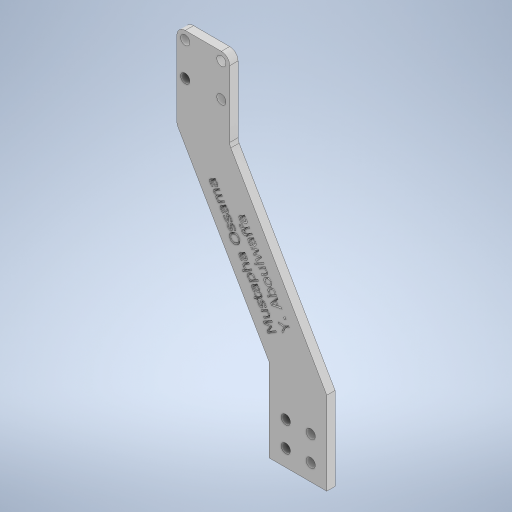
# Autodesk Inventor part: Arm
Saved by Autodesk Inventor 2023 (Build 270158000, 158)
## iProperties
Created: 2023-12-17
Part Number: Arm
Material: Generic
Document SubType Name: Modeling
Designer: Mustapha
Density: 1 g/cm^3
Appearance: Default
Author: Mustapha
Autodesk Inventor part; units mm, degrees
ref_plane "YZ Plane" through (0, 0, 0) normal (1, 0, 0) x (0, 1, 0)
ref_plane "XZ Plane" through (0, 0, 0) normal (0, 1, 0) x (-1, 0, 0)
ref_plane "XY Plane" through (0, 0, 0) normal (0, 0, 1) x (1, 0, 0)
sketch "Sketch1" plane through (0, 0, 0) normal (0, 0, 1) x (1, 0, 0)
  line L0 (0, 0) -> (-54.8483, 95)
  line L1 (-55.5181, 97.5) -> (-55.5181, 142.5)
  line L2 (-50.5181, 147.5) -> (-28.7639, 147.5)
  line L3 (-23.7639, 142.5) -> (-23.7639, 102.5)
  line L4 (-23.094, 100) -> (34.641, 0)
  line L5 (34.641, 0) -> (0, 0)
  arc A0 (-55.5181, 97.5) -> (-54.8483, 95) centre (-50.5181, 97.5) ccw
  arc A1 (-23.7639, 102.5) -> (-23.094, 100) centre (-18.7639, 102.5) ccw
  arc A2 (-23.7639, 142.5) -> (-28.7639, 147.5) centre (-28.7639, 142.5) ccw
  arc A3 (-50.5181, 147.5) -> (-55.5181, 142.5) centre (-50.5181, 142.5) ccw
  line L6 (0, 0) -> (0, -50)
  line L7 (0, -50) -> (34.641, -50)
  line L8 (34.641, -50) -> (34.641, 0)
  circle A4 centre (10, -40) radius 2.75
  circle A5 centre (25, -40) radius 2.75
  circle A6 centre (25, -25) radius 2.75
  circle A7 centre (10, -25) radius 2.75
  circle A8 centre (-50.5181, 142.5) radius 2.75
  circle A9 centre (-28.7639, 142.5) radius 2.75
  circle A10 centre (-50.5181, 122.5) radius 2.75
  circle A11 centre (-28.7639, 122.5) radius 2.75
  point P0 (-55.5181, 147.5)
  dimension "d0" = 5
  dimension "d1" = 30
  dimension "d2" = 50
  dimension "d3" = 5
  dimension "d4" = 50
  dimension "d5" = 40
  dimension "d6" = 100
  dimension "d7" = 120
  dimension "d8" = 5.5
  dimension "d11" = 15
  dimension "d18" = 15
  dimension "d23" = 10
  dimension "d24" = 10
  dimension "d25" = 5.5
  dimension "d26" = 5.5
  dimension "d29" = 20
  constraints: 18 end point, 12 centre point, 8 point on circle, 8 tangent, 5 perpendicular, 4 vertical, 2 coincident, 2 equal radius, 2 point on line, 1 horizontal, 1 parallel, 10 other
  measures "d0" radius of A0
  measures "d1" distance between parallel lines of L0 L4
  measures "d2" distance of L1.start point (-55.518, 147.5)
  measures "d3" radius of A2
  measures "d4" distance of L7.end L4.end
  measures "d5" distance of L3.start L3.end
  measures "d6" vertical distance of L4.start L4.end
  measures "d7" angle of L5 L0
  measures "d8" diameter of A4
  measures "d11" distance of A4.centre A5.centre
  measures "d18" distance of A5.centre A6.centre
  measures "d23" distance from line of L6 A7.centre
  measures "d24" distance from line of L7 A4.centre
  measures "d25" diameter of A8
  measures "d26" diameter of A9
  measures "d29" distance of A8.centre A10.centre
extrude "Extrusion1" add sketch "Sketch1" along normal blind 5
sketch "Sketch2" plane through (0, 0, 5) normal (0, 0, 1) x (1, 0, 0)
  line L0 (-0.614, 13.88) -> (-77.0258, 141.9094) construction
  line L1 (-77.0258, 141.9094) -> (-33.2435, 168.0399) construction
  line L2 (-33.2435, 168.0399) -> (43.1682, 40.0105) construction
  line L3 (43.1682, 40.0105) -> (-0.614, 13.88) construction
  line L4 (1.5283, 22.5197) -> (1.9769, 21.7682)
  line L5 (1.9769, 21.7682) -> (-2.4613, 19.1193)
  line L6 (-2.4613, 19.1193) -> (1.4369, 19.4471)
  line L7 (1.4369, 19.4471) -> (1.7085, 18.992)
  line L8 (1.7085, 18.992) -> (-0.4355, 15.7249)
  line L9 (-0.4355, 15.7249) -> (4.0027, 18.3738)
  line L10 (4.0027, 18.3738) -> (4.4239, 17.6681)
  line L11 (4.4239, 17.6681) -> (-0.7283, 14.5932)
  line L12 (-0.7283, 14.5932) -> (-1.3413, 15.6203)
  line L13 (-1.3413, 15.6203) -> (0.6823, 18.7476)
  line L14 (0.6823, 18.7476) -> (-3.0009, 18.4009)
  line L15 (-3.0009, 18.4009) -> (-3.6238, 19.4447)
  line L16 (-3.6238, 19.4447) -> (1.5283, 22.5197)
  line L17 (-1.1006, 26.9245) -> (-0.6745, 26.2105)
  line L18 (-0.6745, 26.2105) -> (-1.1004, 25.9564)
  spline S0 degree 2 poles (-1.1004, 25.9564) (-0.6405, 25.7835) (-0.0127, 25.3484) (0.2041, 24.9852) knots 0 0 0 1 2 2 2
  spline S1 degree 2 poles (0.2041, 24.9852) (0.371, 24.7055) (0.4956, 24.1173) (0.4257, 23.8264) knots 0 0 0 1 2 2 2
  spline S2 degree 2 poles (0.4257, 23.8264) (0.3558, 23.5356) (-0.0716, 23.0087) (-0.464, 22.7745) knots 0 0 0 1 2 2 2
  line L19 (-0.464, 22.7745) -> (-2.9733, 21.2769)
  line L20 (-2.9733, 21.2769) -> (-3.3994, 21.9908)
  line L21 (-3.3994, 21.9908) -> (-1.1949, 23.3065)
  spline S3 degree 2 poles (-1.1949, 23.3065) (-0.886, 23.4909) (-0.5109, 23.7828) (-0.4129, 23.9601) knots 0 0 0 1 2 2 2
  spline S4 degree 2 poles (-0.4129, 23.9601) (-0.3149, 24.1375) (-0.3566, 24.5204) (-0.5235, 24.8001) knots 0 0 0 1 2 2 2
  spline S5 degree 2 poles (-0.5235, 24.8001) (-0.6805, 25.0631) (-1.3082, 25.4982) (-1.6515, 25.6274) knots 0 0 0 1 2 2 2
  line L22 (-1.6515, 25.6274) -> (-4.5407, 23.9031)
  line L23 (-4.5407, 23.9031) -> (-4.9668, 24.617)
  line L24 (-4.9668, 24.617) -> (-1.1006, 26.9245)
  spline S6 degree 2 poles (-2.312, 29.1629) (-2.0578, 28.737) (-1.823, 27.8693) (-1.7954, 27.5573) knots 0 0 0 1 2 2 2
  line L25 (-1.7954, 27.5573) -> (-2.526, 27.1213)
  line L26 (-2.526, 27.1213) -> (-2.5485, 27.1588)
  spline S7 degree 2 poles (-2.5485, 27.1588) (-2.5365, 27.2906) (-2.5249, 27.6316) (-2.5593, 27.8885) knots 0 0 0 1 2 2 2
  spline S8 degree 2 poles (-2.5593, 27.8885) (-2.5896, 28.1196) (-2.7343, 28.6277) (-2.8739, 28.8615) knots 0 0 0 1 2 2 2
  spline S9 degree 2 poles (-2.8739, 28.8615) (-2.976, 29.0327) (-3.2829, 29.3762) (-3.3945, 29.4398) knots 0 0 0 1 2 2 2
  spline S10 degree 2 poles (-3.3945, 29.4398) (-3.5536, 29.526) (-3.8029, 29.5358) (-3.9866, 29.4262) knots 0 0 0 1 2 2 2
  spline S11 degree 2 poles (-3.9866, 29.4262) (-4.2204, 29.2866) (-4.2898, 28.8715) (-4.1573, 28.4693) knots 0 0 0 1 2 2 2
  spline S12 degree 2 poles (-4.1573, 28.4693) (-4.1085, 28.3116) (-3.9261, 27.8258) (-3.8599, 27.6105) knots 0 0 0 1 2 2 2
  spline S13 degree 2 poles (-3.8599, 27.6105) (-3.7003, 27.049) (-3.9706, 26.2874) (-4.3547, 26.0582) knots 0 0 0 1 2 2 2
  spline S14 degree 2 poles (-4.3547, 26.0582) (-4.8766, 25.7467) (-6.0504, 26.2239) (-6.479, 26.942) knots 0 0 0 1 2 2 2
  spline S15 degree 2 poles (-6.479, 26.942) (-6.6883, 27.2928) (-6.9583, 28.1056) (-6.9817, 28.42) knots 0 0 0 1 2 2 2
  line L27 (-6.9817, 28.42) -> (-6.2845, 28.8361)
  line L28 (-6.2845, 28.8361) -> (-6.262, 28.7986)
  spline S16 degree 2 poles (-6.262, 28.7986) (-6.298, 28.4034) (-6.1264, 27.5941) (-5.9221, 27.2518) knots 0 0 0 1 2 2 2
  spline S17 degree 2 poles (-5.9221, 27.2518) (-5.7128, 26.9011) (-5.1498, 26.5745) (-4.8785, 26.7365) knots 0 0 0 1 2 2 2
  spline S18 degree 2 poles (-4.8785, 26.7365) (-4.6321, 26.8835) (-4.5661, 27.3137) (-4.6803, 27.6758) knots 0 0 0 1 2 2 2
  spline S19 degree 2 poles (-4.6803, 27.6758) (-4.7399, 27.8611) (-4.8965, 28.2942) (-4.9802, 28.5387) knots 0 0 0 1 2 2 2
  spline S20 degree 2 poles (-4.9802, 28.5387) (-5.1532, 29.0753) (-4.9404, 29.8478) (-4.5104, 30.1045) knots 0 0 0 1 2 2 2
  spline S21 degree 2 poles (-4.5104, 30.1045) (-4.2599, 30.254) (-3.6877, 30.301) (-3.4003, 30.1894) knots 0 0 0 1 2 2 2
  spline S22 degree 2 poles (-3.4003, 30.1894) (-3.0921, 30.062) (-2.5711, 29.5971) (-2.312, 29.1629) knots 0 0 0 1 2 2 2
  spline S23 degree 2 poles (-4.4866, 32.7686) (-4.1378, 32.1841) (-4.3519, 31.1673) (-5.0075, 30.7761) knots 0 0 0 1 2 2 2
  line L29 (-5.0075, 30.7761) -> (-7.1493, 29.4977)
  line L30 (-7.1493, 29.4977) -> (-6.8603, 29.0134)
  line L31 (-6.8603, 29.0134) -> (-7.3988, 28.692)
  line L32 (-7.3988, 28.692) -> (-7.6879, 29.1763)
  line L33 (-7.6879, 29.1763) -> (-8.7985, 28.5135)
  line L34 (-8.7985, 28.5135) -> (-9.2246, 29.2274)
  line L35 (-9.2246, 29.2274) -> (-8.114, 29.8903)
  line L36 (-8.114, 29.8903) -> (-8.8989, 31.2054)
  line L37 (-8.8989, 31.2054) -> (-8.3604, 31.5269)
  line L38 (-8.3604, 31.5269) -> (-7.5754, 30.2117)
  line L39 (-7.5754, 30.2117) -> (-5.7342, 31.3106)
  spline S24 degree 2 poles (-5.7342, 31.3106) (-5.4419, 31.485) (-5.1329, 31.6978) (-5.0424, 31.8594) knots 0 0 0 1 2 2 2
  spline S25 degree 2 poles (-5.0424, 31.8594) (-4.9587, 31.9942) (-5.0096, 32.3546) (-5.1591, 32.6051) knots 0 0 0 1 2 2 2
  spline S26 degree 2 poles (-5.1591, 32.6051) (-5.2613, 32.7763) (-5.5542, 33.0488) (-5.6258, 33.1023) knots 0 0 0 1 2 2 2
  line L40 (-5.6258, 33.1023) -> (-5.6507, 33.1441)
  line L41 (-5.6507, 33.1441) -> (-5.0661, 33.493)
  spline S27 degree 2 poles (-5.0661, 33.493) (-4.8964, 33.3225) (-4.5913, 32.944) (-4.4866, 32.7686) knots 0 0 0 1 2 2 2
  spline S28 degree 2 poles (-7.1713, 36.1663) (-7.0605, 36.1135) (-6.6773, 35.9458) (-6.5324, 35.8454) knots 0 0 0 1 2 2 2
  spline S29 degree 2 poles (-6.5324, 35.8454) (-6.3284, 35.7123) (-6.0206, 35.4148) (-5.8312, 35.0974) knots 0 0 0 1 2 2 2
  spline S30 degree 2 poles (-5.8312, 35.0974) (-5.6742, 34.8344) (-5.5722, 34.2555) (-5.6279, 33.9787) knots 0 0 0 1 2 2 2
  spline S31 degree 2 poles (-5.6279, 33.9787) (-5.6844, 33.7129) (-6.0299, 33.2292) (-6.2887, 33.0747) knots 0 0 0 1 2 2 2
  spline S32 degree 2 poles (-6.2887, 33.0747) (-6.6896, 32.8355) (-7.4792, 32.8682) (-7.8837, 33.176) knots 0 0 0 1 2 2 2
  spline S33 degree 2 poles (-7.8837, 33.176) (-8.2458, 33.4412) (-8.9391, 34.3467) (-9.3048, 34.8929) knots 0 0 0 1 2 2 2
  line L42 (-9.3048, 34.8929) -> (-9.43, 34.8182)
  spline S34 degree 2 poles (-9.43, 34.8182) (-9.6555, 34.6836) (-9.8455, 34.3663) (-9.8426, 34.1812) knots 0 0 0 1 2 2 2
  spline S35 degree 2 poles (-9.8426, 34.1812) (-9.8397, 33.9961) (-9.6531, 33.5695) (-9.5285, 33.3608) knots 0 0 0 1 2 2 2
  spline S36 degree 2 poles (-9.5285, 33.3608) (-9.3815, 33.1144) (-8.8492, 32.5262) (-8.5204, 32.2694) knots 0 0 0 1 2 2 2
  line L43 (-8.5204, 32.2694) -> (-8.4955, 32.2276)
  line L44 (-8.4955, 32.2276) -> (-9.1593, 31.8314)
  spline S37 degree 2 poles (-9.1593, 31.8314) (-9.3265, 31.9978) (-9.8929, 32.662) (-10.1096, 33.0253) knots 0 0 0 1 2 2 2
  spline S38 degree 2 poles (-10.1096, 33.0253) (-10.3688, 33.4595) (-10.6024, 34.1355) (-10.5841, 34.4748) knots 0 0 0 1 2 2 2
  spline S39 degree 2 poles (-10.5841, 34.4748) (-10.5625, 34.7991) (-10.1943, 35.3303) (-9.8311, 35.5471) knots 0 0 0 1 2 2 2
  line L45 (-9.8311, 35.5471) -> (-7.1882, 37.1244)
  line L46 (-7.1882, 37.1244) -> (-6.7621, 36.4105)
  line L47 (-6.7621, 36.4105) -> (-7.1713, 36.1663)
  line L48 (-7.714, 35.8423) -> (-8.7871, 35.2019)
  spline S40 degree 2 poles (-8.7871, 35.2019) (-8.6142, 34.9597) (-8.0797, 34.2255) (-7.8684, 34.0232) knots 0 0 0 1 2 2 2
  spline S41 degree 2 poles (-7.8684, 34.0232) (-7.6196, 33.7866) (-7.068, 33.6119) (-6.7757, 33.7863) knots 0 0 0 1 2 2 2
  spline S42 degree 2 poles (-6.7757, 33.7863) (-6.4417, 33.9856) (-6.3477, 34.5967) (-6.5845, 34.9933) knots 0 0 0 1 2 2 2
  spline S43 degree 2 poles (-6.5845, 34.9933) (-6.7863, 35.3315) (-7.3758, 35.7214) (-7.714, 35.8423) knots 0 0 0 1 2 2 2
  spline S44 degree 2 poles (-11.9518, 40.476) (-10.9831, 41.0541) (-9.2336, 40.7223) (-8.7701, 39.9457) knots 0 0 0 1 2 2 2
  spline S45 degree 2 poles (-8.7701, 39.9457) (-8.5833, 39.6326) (-8.4253, 39.0644) (-8.4111, 38.7275) knots 0 0 0 1 2 2 2
  line L49 (-8.4111, 38.7275) -> (-6.7911, 39.6943)
  line L50 (-6.7911, 39.6943) -> (-6.365, 38.9803)
  line L51 (-6.365, 38.9803) -> (-11.6549, 35.8232)
  line L52 (-11.6549, 35.8232) -> (-12.0811, 36.5371)
  line L53 (-12.0811, 36.5371) -> (-11.6761, 36.7788)
  spline S46 degree 2 poles (-11.6761, 36.7788) (-12.0568, 36.914) (-12.7353, 37.3867) (-12.9646, 37.7708) knots 0 0 0 1 2 2 2
  spline S47 degree 2 poles (-12.9646, 37.7708) (-13.4007, 38.5015) (-12.8369, 39.9477) (-11.9518, 40.476) knots 0 0 0 1 2 2 2
  spline S48 degree 2 poles (-11.4356, 39.7819) (-12.0994, 39.3856) (-12.5535, 38.4861) (-12.242, 37.9642) knots 0 0 0 1 2 2 2
  spline S49 degree 2 poles (-12.242, 37.9642) (-12.0626, 37.6636) (-11.4774, 37.2428) (-11.1333, 37.1028) knots 0 0 0 1 2 2 2
  line L54 (-11.1333, 37.1028) -> (-8.9372, 38.4135)
  spline S50 degree 2 poles (-8.9372, 38.4135) (-8.983, 38.7655) (-9.1304, 39.2211) (-9.2849, 39.48) knots 0 0 0 1 2 2 2
  spline S51 degree 2 poles (-9.2849, 39.48) (-9.6163, 40.0353) (-10.7258, 40.2055) (-11.4356, 39.7819) knots 0 0 0 1 2 2 2
  line L55 (-12.3513, 45.7753) -> (-11.9252, 45.0614)
  line L56 (-11.9252, 45.0614) -> (-14.1297, 43.7457)
  spline S52 degree 2 poles (-14.1297, 43.7457) (-14.3969, 43.5862) (-14.8213, 43.2537) (-14.9117, 43.0921) knots 0 0 0 1 2 2 2
  spline S53 degree 2 poles (-14.9117, 43.0921) (-15.0055, 42.9172) (-14.9606, 42.5193) (-14.8011, 42.2521) knots 0 0 0 1 2 2 2
  spline S54 degree 2 poles (-14.8011, 42.2521) (-14.6417, 41.9849) (-14.0439, 41.5716) (-13.6732, 41.4248) knots 0 0 0 1 2 2 2
  line L57 (-13.6732, 41.4248) -> (-10.784, 43.1492)
  line L58 (-10.784, 43.1492) -> (-10.3579, 42.4352)
  line L59 (-10.3579, 42.4352) -> (-15.7396, 39.2232)
  line L60 (-15.7396, 39.2232) -> (-16.1657, 39.9372)
  line L61 (-16.1657, 39.9372) -> (-14.2201, 41.0984)
  spline S55 degree 2 poles (-14.2201, 41.0984) (-14.675, 41.2629) (-15.3219, 41.7205) (-15.5287, 42.067) knots 0 0 0 1 2 2 2
  spline S56 degree 2 poles (-15.5287, 42.067) (-15.9025, 42.6933) (-15.5746, 43.8516) (-14.8606, 44.2777) knots 0 0 0 1 2 2 2
  line L62 (-14.8606, 44.2777) -> (-12.3513, 45.7753)
  spline S57 degree 2 poles (-14.7739, 48.9047) (-14.6631, 48.8519) (-14.28, 48.6842) (-14.1351, 48.5838) knots 0 0 0 1 2 2 2
  spline S58 degree 2 poles (-14.1351, 48.5838) (-13.9311, 48.4507) (-13.6233, 48.1532) (-13.4339, 47.8359) knots 0 0 0 1 2 2 2
  spline S59 degree 2 poles (-13.4339, 47.8359) (-13.2769, 47.5728) (-13.1749, 46.9939) (-13.2305, 46.7172) knots 0 0 0 1 2 2 2
  spline S60 degree 2 poles (-13.2305, 46.7172) (-13.287, 46.4513) (-13.6325, 45.9676) (-13.8914, 45.8131) knots 0 0 0 1 2 2 2
  spline S61 degree 2 poles (-13.8914, 45.8131) (-14.2922, 45.5739) (-15.0818, 45.6066) (-15.4864, 45.9144) knots 0 0 0 1 2 2 2
  spline S62 degree 2 poles (-15.4864, 45.9144) (-15.8485, 46.1796) (-16.5418, 47.0851) (-16.9074, 47.6313) knots 0 0 0 1 2 2 2
  line L63 (-16.9074, 47.6313) -> (-17.0327, 47.5566)
  spline S63 degree 2 poles (-17.0327, 47.5566) (-17.2582, 47.422) (-17.4482, 47.1048) (-17.4453, 46.9196) knots 0 0 0 1 2 2 2
  spline S64 degree 2 poles (-17.4453, 46.9196) (-17.4424, 46.7345) (-17.2557, 46.308) (-17.1312, 46.0992) knots 0 0 0 1 2 2 2
  spline S65 degree 2 poles (-17.1312, 46.0992) (-16.9841, 45.8529) (-16.4518, 45.2646) (-16.1231, 45.0078) knots 0 0 0 1 2 2 2
  line L64 (-16.1231, 45.0078) -> (-16.0981, 44.9661)
  line L65 (-16.0981, 44.9661) -> (-16.762, 44.5699)
  spline S66 degree 2 poles (-16.762, 44.5699) (-16.9292, 44.7362) (-17.4955, 45.4004) (-17.7123, 45.7637) knots 0 0 0 1 2 2 2
  spline S67 degree 2 poles (-17.7123, 45.7637) (-17.9715, 46.1979) (-18.205, 46.8739) (-18.1867, 47.2132) knots 0 0 0 1 2 2 2
  spline S68 degree 2 poles (-18.1867, 47.2132) (-18.1651, 47.5375) (-17.797, 48.0687) (-17.4338, 48.2855) knots 0 0 0 1 2 2 2
  line L66 (-17.4338, 48.2855) -> (-14.7909, 49.8628)
  line L67 (-14.7909, 49.8628) -> (-14.3648, 49.1489)
  line L68 (-14.3648, 49.1489) -> (-14.7739, 48.9047)
  line L69 (-15.3167, 48.5807) -> (-16.3897, 47.9403)
  spline S69 degree 2 poles (-16.3897, 47.9403) (-16.2168, 47.6981) (-15.6824, 46.9639) (-15.471, 46.7616) knots 0 0 0 1 2 2 2
  spline S70 degree 2 poles (-15.471, 46.7616) (-15.2223, 46.525) (-14.6707, 46.3503) (-14.3784, 46.5247) knots 0 0 0 1 2 2 2
  spline S71 degree 2 poles (-14.3784, 46.5247) (-14.0444, 46.7241) (-13.9504, 47.3351) (-14.1871, 47.7317) knots 0 0 0 1 2 2 2
  spline S72 degree 2 poles (-14.1871, 47.7317) (-14.389, 48.0699) (-14.9784, 48.4599) (-15.3167, 48.5807) knots 0 0 0 1 2 2 2
  spline S73 degree 2 poles (-23.8322, 54.642) (-23.6817, 55.1678) (-22.894, 56.1249) (-22.251, 56.5087) knots 0 0 0 1 2 2 2
  spline S74 degree 2 poles (-22.251, 56.5087) (-21.6247, 56.8824) (-20.4008, 57.1373) (-19.8616, 57.0117) knots 0 0 0 1 2 2 2
  spline S75 degree 2 poles (-19.8616, 57.0117) (-19.2957, 56.8795) (-18.4027, 56.1611) (-18.0712, 55.6058) knots 0 0 0 1 2 2 2
  spline S76 degree 2 poles (-18.0712, 55.6058) (-17.7274, 55.0297) (-17.5316, 53.8951) (-17.6812, 53.3585) knots 0 0 0 1 2 2 2
  spline S77 degree 2 poles (-17.6812, 53.3585) (-17.8292, 52.8285) (-18.6261, 51.8772) (-19.2608, 51.4985) knots 0 0 0 1 2 2 2
  spline S78 degree 2 poles (-19.2608, 51.4985) (-19.9079, 51.1122) (-21.1051, 50.879) (-21.6543, 50.9929) knots 0 0 0 1 2 2 2
  spline S79 degree 2 poles (-21.6543, 50.9929) (-22.191, 51.1142) (-23.0991, 51.8293) (-23.4405, 52.4013) knots 0 0 0 1 2 2 2
  spline S80 degree 2 poles (-23.4405, 52.4013) (-23.7844, 52.9775) (-23.9702, 54.1236) (-23.8322, 54.642) knots 0 0 0 1 2 2 2
  spline S81 degree 2 poles (-21.7825, 55.7237) (-22.2919, 55.4197) (-22.9365, 54.7066) (-23.0633, 54.3308) knots 0 0 0 1 2 2 2
  spline S82 degree 2 poles (-23.0633, 54.3308) (-23.1959, 53.9459) (-23.0844, 53.1518) (-22.8476, 52.7551) knots 0 0 0 1 2 2 2
  spline S83 degree 2 poles (-22.8476, 52.7551) (-22.6034, 52.346) (-21.9808, 51.8909) (-21.5632, 51.8174) knots 0 0 0 1 2 2 2
  spline S84 degree 2 poles (-21.5632, 51.8174) (-21.1656, 51.7489) (-20.2303, 51.9844) (-19.7292, 52.2834) knots 0 0 0 1 2 2 2
  spline S85 degree 2 poles (-19.7292, 52.2834) (-18.7147, 52.8889) (-18.1957, 54.4671) (-18.6641, 55.252) knots 0 0 0 1 2 2 2
  spline S86 degree 2 poles (-18.6641, 55.252) (-19.1351, 56.0411) (-20.768, 56.3293) (-21.7825, 55.7237) knots 0 0 0 1 2 2 2
  spline S87 degree 2 poles (-20.7268, 60.0174) (-20.4727, 59.5915) (-20.2379, 58.7237) (-20.2102, 58.4118) knots 0 0 0 1 2 2 2
  line L70 (-20.2102, 58.4118) -> (-20.9409, 57.9757)
  line L71 (-20.9409, 57.9757) -> (-20.9633, 58.0133)
  spline S88 degree 2 poles (-20.9633, 58.0133) (-20.9513, 58.145) (-20.9397, 58.486) (-20.9741, 58.743) knots 0 0 0 1 2 2 2
  spline S89 degree 2 poles (-20.9741, 58.743) (-21.0044, 58.974) (-21.1492, 59.4822) (-21.2887, 59.716) knots 0 0 0 1 2 2 2
  spline S90 degree 2 poles (-21.2887, 59.716) (-21.3909, 59.8872) (-21.6978, 60.2306) (-21.8094, 60.2942) knots 0 0 0 1 2 2 2
  spline S91 degree 2 poles (-21.8094, 60.2942) (-21.9684, 60.3805) (-22.2177, 60.3902) (-22.4015, 60.2806) knots 0 0 0 1 2 2 2
  spline S92 degree 2 poles (-22.4015, 60.2806) (-22.6353, 60.1411) (-22.7046, 59.726) (-22.5721, 59.3237) knots 0 0 0 1 2 2 2
  spline S93 degree 2 poles (-22.5721, 59.3237) (-22.5233, 59.166) (-22.341, 58.6803) (-22.2748, 58.465) knots 0 0 0 1 2 2 2
  spline S94 degree 2 poles (-22.2748, 58.465) (-22.1152, 57.9034) (-22.3854, 57.1419) (-22.7696, 56.9126) knots 0 0 0 1 2 2 2
  spline S95 degree 2 poles (-22.7696, 56.9126) (-23.2914, 56.6012) (-24.4653, 57.0784) (-24.8939, 57.7965) knots 0 0 0 1 2 2 2
  spline S96 degree 2 poles (-24.8939, 57.7965) (-25.1032, 58.1472) (-25.3731, 58.96) (-25.3966, 59.2744) knots 0 0 0 1 2 2 2
  line L72 (-25.3966, 59.2744) -> (-24.6993, 59.6906)
  line L73 (-24.6993, 59.6906) -> (-24.6769, 59.653)
  spline S97 degree 2 poles (-24.6769, 59.653) (-24.7128, 59.2578) (-24.5413, 58.4486) (-24.3369, 58.1062) knots 0 0 0 1 2 2 2
  spline S98 degree 2 poles (-24.3369, 58.1062) (-24.1276, 57.7555) (-23.5647, 57.429) (-23.2933, 57.591) knots 0 0 0 1 2 2 2
  spline S99 degree 2 poles (-23.2933, 57.591) (-23.047, 57.738) (-22.9809, 58.1681) (-23.0952, 58.5303) knots 0 0 0 1 2 2 2
  spline S100 degree 2 poles (-23.0952, 58.5303) (-23.1548, 58.7155) (-23.3113, 59.1487) (-23.395, 59.3932) knots 0 0 0 1 2 2 2
  spline S101 degree 2 poles (-23.395, 59.3932) (-23.568, 59.9298) (-23.3553, 60.7023) (-22.9252, 60.9589) knots 0 0 0 1 2 2 2
  spline S102 degree 2 poles (-22.9252, 60.9589) (-22.6747, 61.1084) (-22.1026, 61.1555) (-21.8151, 61.0439) knots 0 0 0 1 2 2 2
  spline S103 degree 2 poles (-21.8151, 61.0439) (-21.5069, 60.9164) (-20.986, 60.4516) (-20.7268, 60.0174) knots 0 0 0 1 2 2 2
  spline S104 degree 2 poles (-22.8025, 63.4953) (-22.5484, 63.0694) (-22.3136, 62.2016) (-22.286, 61.8897) knots 0 0 0 1 2 2 2
  line L74 (-22.286, 61.8897) -> (-23.0166, 61.4536)
  line L75 (-23.0166, 61.4536) -> (-23.039, 61.4912)
  spline S105 degree 2 poles (-23.039, 61.4912) (-23.0271, 61.6229) (-23.0154, 61.964) (-23.0498, 62.2209) knots 0 0 0 1 2 2 2
  spline S106 degree 2 poles (-23.0498, 62.2209) (-23.0802, 62.4519) (-23.2249, 62.9601) (-23.3644, 63.1939) knots 0 0 0 1 2 2 2
  spline S107 degree 2 poles (-23.3644, 63.1939) (-23.4666, 63.3651) (-23.7735, 63.7085) (-23.8851, 63.7721) knots 0 0 0 1 2 2 2
  spline S108 degree 2 poles (-23.8851, 63.7721) (-24.0442, 63.8584) (-24.2935, 63.8682) (-24.4772, 63.7585) knots 0 0 0 1 2 2 2
  spline S109 degree 2 poles (-24.4772, 63.7585) (-24.711, 63.619) (-24.7803, 63.2039) (-24.6479, 62.8016) knots 0 0 0 1 2 2 2
  spline S110 degree 2 poles (-24.6479, 62.8016) (-24.599, 62.6439) (-24.4167, 62.1582) (-24.3505, 61.9429) knots 0 0 0 1 2 2 2
  spline S111 degree 2 poles (-24.3505, 61.9429) (-24.1909, 61.3813) (-24.4612, 60.6198) (-24.8453, 60.3905) knots 0 0 0 1 2 2 2
  spline S112 degree 2 poles (-24.8453, 60.3905) (-25.3672, 60.0791) (-26.541, 60.5563) (-26.9696, 61.2744) knots 0 0 0 1 2 2 2
  spline S113 degree 2 poles (-26.9696, 61.2744) (-27.1789, 61.6251) (-27.4488, 62.4379) (-27.4723, 62.7524) knots 0 0 0 1 2 2 2
  line L76 (-27.4723, 62.7524) -> (-26.775, 63.1685)
  line L77 (-26.775, 63.1685) -> (-26.7526, 63.1309)
  spline S114 degree 2 poles (-26.7526, 63.1309) (-26.7885, 62.7358) (-26.617, 61.9265) (-26.4127, 61.5841) knots 0 0 0 1 2 2 2
  spline S115 degree 2 poles (-26.4127, 61.5841) (-26.2033, 61.2334) (-25.6404, 60.9069) (-25.369, 61.0689) knots 0 0 0 1 2 2 2
  spline S116 degree 2 poles (-25.369, 61.0689) (-25.1227, 61.2159) (-25.0566, 61.646) (-25.1709, 62.0082) knots 0 0 0 1 2 2 2
  spline S117 degree 2 poles (-25.1709, 62.0082) (-25.2305, 62.1934) (-25.3871, 62.6266) (-25.4707, 62.8711) knots 0 0 0 1 2 2 2
  spline S118 degree 2 poles (-25.4707, 62.8711) (-25.6437, 63.4077) (-25.431, 64.1802) (-25.0009, 64.4368) knots 0 0 0 1 2 2 2
  spline S119 degree 2 poles (-25.0009, 64.4368) (-24.7504, 64.5864) (-24.1783, 64.6334) (-23.8909, 64.5218) knots 0 0 0 1 2 2 2
  spline S120 degree 2 poles (-23.8909, 64.5218) (-23.5826, 64.3943) (-23.0617, 63.9295) (-22.8025, 63.4953) knots 0 0 0 1 2 2 2
  spline S121 degree 2 poles (-26.1069, 67.8933) (-25.9961, 67.8405) (-25.6129, 67.6728) (-25.4681, 67.5724) knots 0 0 0 1 2 2 2
  spline S122 degree 2 poles (-25.4681, 67.5724) (-25.2641, 67.4394) (-24.9563, 67.1418) (-24.7669, 66.8245) knots 0 0 0 1 2 2 2
  spline S123 degree 2 poles (-24.7669, 66.8245) (-24.6099, 66.5615) (-24.5078, 65.9825) (-24.5635, 65.7058) knots 0 0 0 1 2 2 2
  spline S124 degree 2 poles (-24.5635, 65.7058) (-24.62, 65.4399) (-24.9655, 64.9563) (-25.2244, 64.8018) knots 0 0 0 1 2 2 2
  spline S125 degree 2 poles (-25.2244, 64.8018) (-25.6252, 64.5625) (-26.4148, 64.5952) (-26.8193, 64.9031) knots 0 0 0 1 2 2 2
  spline S126 degree 2 poles (-26.8193, 64.9031) (-27.1815, 65.1682) (-27.8748, 66.0738) (-28.2404, 66.62) knots 0 0 0 1 2 2 2
  line L78 (-28.2404, 66.62) -> (-28.3657, 66.5452)
  spline S127 degree 2 poles (-28.3657, 66.5452) (-28.5911, 66.4107) (-28.7812, 66.0934) (-28.7783, 65.9083) knots 0 0 0 1 2 2 2
  spline S128 degree 2 poles (-28.7783, 65.9083) (-28.7754, 65.7231) (-28.5887, 65.2966) (-28.4641, 65.0878) knots 0 0 0 1 2 2 2
  spline S129 degree 2 poles (-28.4641, 65.0878) (-28.3171, 64.8415) (-27.7848, 64.2532) (-27.456, 63.9965) knots 0 0 0 1 2 2 2
  line L79 (-27.456, 63.9965) -> (-27.4311, 63.9547)
  line L80 (-27.4311, 63.9547) -> (-28.095, 63.5585)
  spline S130 degree 2 poles (-28.095, 63.5585) (-28.2622, 63.7248) (-28.8285, 64.3891) (-29.0453, 64.7523) knots 0 0 0 1 2 2 2
  spline S131 degree 2 poles (-29.0453, 64.7523) (-29.3044, 65.1865) (-29.538, 65.8625) (-29.5197, 66.2019) knots 0 0 0 1 2 2 2
  spline S132 degree 2 poles (-29.5197, 66.2019) (-29.4981, 66.5262) (-29.13, 67.0573) (-28.7667, 67.2741) knots 0 0 0 1 2 2 2
  line L81 (-28.7667, 67.2741) -> (-26.1239, 68.8515)
  line L82 (-26.1239, 68.8515) -> (-25.6977, 68.1375)
  line L83 (-25.6977, 68.1375) -> (-26.1069, 67.8933)
  line L84 (-26.6497, 67.5694) -> (-27.7227, 66.929)
  spline S133 degree 2 poles (-27.7227, 66.929) (-27.5498, 66.6867) (-27.0154, 65.9525) (-26.804, 65.7502) knots 0 0 0 1 2 2 2
  spline S134 degree 2 poles (-26.804, 65.7502) (-26.5552, 65.5137) (-26.0036, 65.3389) (-25.7114, 65.5134) knots 0 0 0 1 2 2 2
  spline S135 degree 2 poles (-25.7114, 65.5134) (-25.3774, 65.7127) (-25.2834, 66.3237) (-25.5201, 66.7204) knots 0 0 0 1 2 2 2
  spline S136 degree 2 poles (-25.5201, 66.7204) (-25.7219, 67.0585) (-26.3114, 67.4485) (-26.6497, 67.5694) knots 0 0 0 1 2 2 2
  line L85 (-29.605, 74.6842) -> (-31.8429, 73.3485)
  spline S137 degree 2 poles (-31.8429, 73.3485) (-32.1101, 73.189) (-32.5378, 72.8715) (-32.6207, 72.7258) knots 0 0 0 1 2 2 2
  spline S138 degree 2 poles (-32.6207, 72.7258) (-32.7111, 72.5642) (-32.6777, 72.2047) (-32.5332, 71.9626) knots 0 0 0 1 2 2 2
  spline S139 degree 2 poles (-32.5332, 71.9626) (-32.4036, 71.7455) (-31.8533, 71.3831) (-31.4575, 71.2513) knots 0 0 0 1 2 2 2
  spline S140 degree 2 poles (-31.4575, 71.2513) (-31.4016, 71.2903) (-31.2462, 71.4001) (-31.1376, 71.4648) knots 0 0 0 1 2 2 2
  line L86 (-31.1376, 71.4648) -> (-28.5908, 72.9849)
  line L87 (-28.5908, 72.9849) -> (-28.1647, 72.2709)
  line L88 (-28.1647, 72.2709) -> (-30.4026, 70.9353)
  spline S141 degree 2 poles (-30.4026, 70.9353) (-30.6698, 70.7758) (-31.0975, 70.4583) (-31.1804, 70.3125) knots 0 0 0 1 2 2 2
  spline S142 degree 2 poles (-31.1804, 70.3125) (-31.2708, 70.151) (-31.2374, 69.7915) (-31.0929, 69.5493) knots 0 0 0 1 2 2 2
  spline S143 degree 2 poles (-31.0929, 69.5493) (-30.9559, 69.3197) (-30.3863, 68.9631) (-30.0397, 68.8473) knots 0 0 0 1 2 2 2
  line L89 (-30.0397, 68.8473) -> (-27.1505, 70.5716)
  line L90 (-27.1505, 70.5716) -> (-26.7244, 69.8577)
  line L91 (-26.7244, 69.8577) -> (-30.5906, 67.5502)
  line L92 (-30.5906, 67.5502) -> (-31.0167, 68.2642)
  line L93 (-31.0167, 68.2642) -> (-30.5908, 68.5183)
  spline S144 degree 2 poles (-30.5908, 68.5183) (-31.0125, 68.6461) (-31.6236, 69.0344) (-31.8205, 69.3643) knots 0 0 0 1 2 2 2
  spline S145 degree 2 poles (-31.8205, 69.3643) (-32.0447, 69.74) (-32.0805, 70.5114) (-31.8153, 70.8735) knots 0 0 0 1 2 2 2
  spline S146 degree 2 poles (-31.8153, 70.8735) (-32.3395, 71.0023) (-33.044, 71.4143) (-33.2608, 71.7775) knots 0 0 0 1 2 2 2
  spline S147 degree 2 poles (-33.2608, 71.7775) (-33.4252, 72.0531) (-33.5374, 72.592) (-33.4617, 72.8637) knots 0 0 0 1 2 2 2
  spline S148 degree 2 poles (-33.4617, 72.8637) (-33.3885, 73.1395) (-32.9746, 73.6414) (-32.5779, 73.8781) knots 0 0 0 1 2 2 2
  line L94 (-32.5779, 73.8781) -> (-30.0311, 75.3981)
  line L95 (-30.0311, 75.3981) -> (-29.605, 74.6842)
  spline S149 degree 2 poles (-32.4512, 78.5233) (-32.3404, 78.4705) (-31.9572, 78.3028) (-31.8124, 78.2024) knots 0 0 0 1 2 2 2
  spline S150 degree 2 poles (-31.8124, 78.2024) (-31.6084, 78.0693) (-31.3005, 77.7718) (-31.1112, 77.4545) knots 0 0 0 1 2 2 2
  spline S151 degree 2 poles (-31.1112, 77.4545) (-30.9542, 77.1914) (-30.8521, 76.6125) (-30.9078, 76.3358) knots 0 0 0 1 2 2 2
  spline S152 degree 2 poles (-30.9078, 76.3358) (-30.9643, 76.0699) (-31.3098, 75.5862) (-31.5687, 75.4317) knots 0 0 0 1 2 2 2
  spline S153 degree 2 poles (-31.5687, 75.4317) (-31.9695, 75.1925) (-32.7591, 75.2252) (-33.1636, 75.533) knots 0 0 0 1 2 2 2
  spline S154 degree 2 poles (-33.1636, 75.533) (-33.5257, 75.7982) (-34.2191, 76.7037) (-34.5847, 77.2499) knots 0 0 0 1 2 2 2
  line L96 (-34.5847, 77.2499) -> (-34.7099, 77.1752)
  spline S155 degree 2 poles (-34.7099, 77.1752) (-34.9354, 77.0406) (-35.1254, 76.7234) (-35.1225, 76.5382) knots 0 0 0 1 2 2 2
  spline S156 degree 2 poles (-35.1225, 76.5382) (-35.1196, 76.3531) (-34.933, 75.9266) (-34.8084, 75.7178) knots 0 0 0 1 2 2 2
  spline S157 degree 2 poles (-34.8084, 75.7178) (-34.6614, 75.4715) (-34.1291, 74.8832) (-33.8003, 74.6264) knots 0 0 0 1 2 2 2
  line L97 (-33.8003, 74.6264) -> (-33.7754, 74.5847)
  line L98 (-33.7754, 74.5847) -> (-34.4392, 74.1885)
  spline S158 degree 2 poles (-34.4392, 74.1885) (-34.6065, 74.3548) (-35.1728, 75.019) (-35.3896, 75.3823) knots 0 0 0 1 2 2 2
  spline S159 degree 2 poles (-35.3896, 75.3823) (-35.6487, 75.8165) (-35.8823, 76.4925) (-35.864, 76.8318) knots 0 0 0 1 2 2 2
  spline S160 degree 2 poles (-35.864, 76.8318) (-35.8424, 77.1561) (-35.4742, 77.6873) (-35.111, 77.9041) knots 0 0 0 1 2 2 2
  line L99 (-35.111, 77.9041) -> (-32.4681, 79.4814)
  line L100 (-32.4681, 79.4814) -> (-32.042, 78.7675)
  line L101 (-32.042, 78.7675) -> (-32.4512, 78.5233)
  line L102 (-32.994, 78.1993) -> (-34.067, 77.5589)
  spline S161 degree 2 poles (-34.067, 77.5589) (-33.8941, 77.3167) (-33.3596, 76.5825) (-33.1483, 76.3802) knots 0 0 0 1 2 2 2
  spline S162 degree 2 poles (-33.1483, 76.3802) (-32.8995, 76.1436) (-32.3479, 75.9689) (-32.0557, 76.1433) knots 0 0 0 1 2 2 2
  spline S163 degree 2 poles (-32.0557, 76.1433) (-31.7216, 76.3427) (-31.6277, 76.9537) (-31.8644, 77.3503) knots 0 0 0 1 2 2 2
  spline S164 degree 2 poles (-31.8644, 77.3503) (-32.0662, 77.6885) (-32.6557, 78.0785) (-32.994, 78.1993) knots 0 0 0 1 2 2 2
  line L103 (5.3923, 23.6141) -> (9.4061, 23.4163)
  line L104 (9.4061, 23.4163) -> (11.6857, 24.7768)
  line L105 (11.6857, 24.7768) -> (12.1343, 24.0253)
  line L106 (12.1343, 24.0253) -> (9.9256, 22.7071)
  line L107 (9.9256, 22.7071) -> (8.1234, 19.0381)
  line L108 (8.1234, 19.0381) -> (7.625, 19.8731)
  line L109 (7.625, 19.8731) -> (9.0242, 22.69)
  line L110 (9.0242, 22.69) -> (5.8683, 22.8166)
  line L111 (5.8683, 22.8166) -> (5.3923, 23.6141)
  line L112 (9.5976, 28.2756) -> (10.1408, 27.3654)
  line L113 (10.1408, 27.3654) -> (9.1554, 26.7773)
  line L114 (9.1554, 26.7773) -> (8.6122, 27.6875)
  line L115 (8.6122, 27.6875) -> (9.5976, 28.2756)
  line L116 (7.7336, 31.3986) -> (1.4427, 30.2317)
  line L117 (1.4427, 30.2317) -> (0.887, 31.1628)
  line L118 (0.887, 31.1628) -> (4.9004, 36.1458)
  line L119 (4.9004, 36.1458) -> (5.3738, 35.3525)
  line L120 (5.3738, 35.3525) -> (4.2399, 33.9793)
  line L121 (4.2399, 33.9793) -> (5.5332, 31.8124)
  line L122 (5.5332, 31.8124) -> (7.2801, 32.1585)
  line L123 (7.2801, 32.1585) -> (7.7336, 31.3986)
  line L124 (3.78, 33.4216) -> (1.8733, 31.0946)
  line L125 (1.8733, 31.0946) -> (4.8216, 31.6764)
  line L126 (4.8216, 31.6764) -> (3.78, 33.4216)
  spline S165 degree 2 poles (0.4925, 38.9962) (1.4403, 39.5619) (3.1999, 39.2417) (3.6534, 38.4819) knots 0 0 0 1 2 2 2
  spline S166 degree 2 poles (3.6534, 38.4819) (3.8602, 38.1353) (3.9998, 37.5504) (4.0082, 37.2327) knots 0 0 0 1 2 2 2
  line L127 (4.0082, 37.2327) -> (4.2151, 37.2939)
  line L128 (4.2151, 37.2939) -> (4.6138, 36.6259)
  line L129 (4.6138, 36.6259) -> (-0.768, 33.4139)
  line L130 (-0.768, 33.4139) -> (-1.1941, 34.1279)
  line L131 (-1.1941, 34.1279) -> (0.7265, 35.2741)
  spline S167 degree 2 poles (0.7265, 35.2741) (0.3433, 35.4134) (-0.3253, 35.8695) (-0.562, 36.2661) knots 0 0 0 1 2 2 2
  spline S168 degree 2 poles (-0.562, 36.2661) (-0.9931, 36.9884) (-0.4385, 38.4405) (0.4925, 38.9962) knots 0 0 0 1 2 2 2
  spline S169 degree 2 poles (0.9837, 38.2871) (0.2906, 37.8735) (-0.1509, 36.9814) (0.1556, 36.4679) knots 0 0 0 1 2 2 2
  spline S170 degree 2 poles (0.1556, 36.4679) (0.33, 36.1756) (0.9369, 35.7281) (1.2735, 35.6006) knots 0 0 0 1 2 2 2
  line L132 (1.2735, 35.6006) -> (3.4905, 36.9237)
  spline S171 degree 2 poles (3.4905, 36.9237) (3.4496, 37.2674) (3.3006, 37.7447) (3.1511, 37.9952) knots 0 0 0 1 2 2 2
  spline S172 degree 2 poles (3.1511, 37.9952) (2.8247, 38.5422) (1.7478, 38.7431) (0.9837, 38.2871) knots 0 0 0 1 2 2 2
  spline S173 degree 2 poles (-1.9741, 43.2714) (-0.9971, 43.8545) (0.6856, 43.4545) (1.1989, 42.5944) knots 0 0 0 1 2 2 2
  spline S174 degree 2 poles (1.1989, 42.5944) (1.7272, 41.7093) (1.2346, 40.0393) (0.291, 39.4762) knots 0 0 0 1 2 2 2
  spline S175 degree 2 poles (0.291, 39.4762) (-0.6776, 38.8981) (-2.3736, 39.3014) (-2.8844, 40.1574) knots 0 0 0 1 2 2 2
  spline S176 degree 2 poles (-2.8844, 40.1574) (-3.3977, 41.0174) (-2.9469, 42.6908) (-1.9741, 43.2714) knots 0 0 0 1 2 2 2
  spline S177 degree 2 poles (-1.533, 42.5324) (-2.2845, 42.0839) (-2.6564, 41.0466) (-2.3249, 40.4913) knots 0 0 0 1 2 2 2
  spline S178 degree 2 poles (-2.3249, 40.4913) (-1.9935, 39.936) (-0.9016, 39.7666) (-0.15, 40.2152) knots 0 0 0 1 2 2 2
  spline S179 degree 2 poles (-0.15, 40.2152) (0.5806, 40.6513) (0.9708, 41.7052) (0.6394, 42.2605) knots 0 0 0 1 2 2 2
  spline S180 degree 2 poles (0.6394, 42.2605) (0.3105, 42.8116) (-0.7898, 42.9759) (-1.533, 42.5324) knots 0 0 0 1 2 2 2
  line L133 (-2.4556, 48.4709) -> (-2.0295, 47.7569)
  line L134 (-2.0295, 47.7569) -> (-2.4553, 47.5027)
  spline S181 degree 2 poles (-2.4553, 47.5027) (-1.9954, 47.3299) (-1.3677, 46.8948) (-1.1509, 46.5316) knots 0 0 0 1 2 2 2
  spline S182 degree 2 poles (-1.1509, 46.5316) (-0.984, 46.2518) (-0.8594, 45.6637) (-0.9293, 45.3728) knots 0 0 0 1 2 2 2
  spline S183 degree 2 poles (-0.9293, 45.3728) (-0.9992, 45.082) (-1.4266, 44.5551) (-1.819, 44.3209) knots 0 0 0 1 2 2 2
  line L135 (-1.819, 44.3209) -> (-4.3283, 42.8233)
  line L136 (-4.3283, 42.8233) -> (-4.7544, 43.5372)
  line L137 (-4.7544, 43.5372) -> (-2.5499, 44.8529)
  spline S184 degree 2 poles (-2.5499, 44.8529) (-2.2409, 45.0373) (-1.8659, 45.3291) (-1.7679, 45.5065) knots 0 0 0 1 2 2 2
  spline S185 degree 2 poles (-1.7679, 45.5065) (-1.6699, 45.6839) (-1.7115, 46.0667) (-1.8785, 46.3465) knots 0 0 0 1 2 2 2
  spline S186 degree 2 poles (-1.8785, 46.3465) (-2.0355, 46.6095) (-2.6632, 47.0446) (-3.0065, 47.1738) knots 0 0 0 1 2 2 2
  line L138 (-3.0065, 47.1738) -> (-5.8957, 45.4494)
  line L139 (-5.8957, 45.4494) -> (-6.3218, 46.1634)
  line L140 (-6.3218, 46.1634) -> (-2.4556, 48.4709)
  line L141 (-3.5071, 50.2328) -> (-3.081, 49.5188)
  line L142 (-3.081, 49.5188) -> (-8.4628, 46.3068)
  line L143 (-8.4628, 46.3068) -> (-8.8889, 47.0208)
  line L144 (-8.8889, 47.0208) -> (-3.5071, 50.2328)
  line L145 (-11.0762, 54.1296) -> (-6.5671, 55.3599)
  line L146 (-6.5671, 55.3599) -> (-6.1709, 54.696)
  line L147 (-6.1709, 54.696) -> (-8.534, 51.8814)
  line L148 (-8.534, 51.8814) -> (-4.935, 52.6251)
  line L149 (-4.935, 52.6251) -> (-4.5438, 51.9696)
  line L150 (-4.5438, 51.9696) -> (-7.7596, 48.5725)
  line L151 (-7.7596, 48.5725) -> (-8.2056, 49.3198)
  line L152 (-8.2056, 49.3198) -> (-5.6581, 51.8538)
  line L153 (-5.6581, 51.8538) -> (-9.2547, 51.0776)
  line L154 (-9.2547, 51.0776) -> (-9.606, 51.6663)
  line L155 (-9.606, 51.6663) -> (-7.2304, 54.4884)
  line L156 (-7.2304, 54.4884) -> (-10.6476, 53.4115)
  line L157 (-10.6476, 53.4115) -> (-11.0762, 54.1296)
  spline S187 degree 2 poles (-9.4084, 59.1906) (-9.2976, 59.1378) (-8.9144, 58.9702) (-8.7695, 58.8698) knots 0 0 0 1 2 2 2
  spline S188 degree 2 poles (-8.7695, 58.8698) (-8.5656, 58.7367) (-8.2577, 58.4391) (-8.0683, 58.1218) knots 0 0 0 1 2 2 2
  spline S189 degree 2 poles (-8.0683, 58.1218) (-7.9113, 57.8588) (-7.8093, 57.2798) (-7.865, 57.0031) knots 0 0 0 1 2 2 2
  spline S190 degree 2 poles (-7.865, 57.0031) (-7.9215, 56.7373) (-8.267, 56.2536) (-8.5258, 56.0991) knots 0 0 0 1 2 2 2
  spline S191 degree 2 poles (-8.5258, 56.0991) (-8.9267, 55.8599) (-9.7163, 55.8926) (-10.1208, 56.2004) knots 0 0 0 1 2 2 2
  spline S192 degree 2 poles (-10.1208, 56.2004) (-10.4829, 56.4656) (-11.1762, 57.3711) (-11.5419, 57.9173) knots 0 0 0 1 2 2 2
  line L158 (-11.5419, 57.9173) -> (-11.6671, 57.8425)
  spline S193 degree 2 poles (-11.6671, 57.8425) (-11.8926, 57.708) (-12.0826, 57.3907) (-12.0797, 57.2056) knots 0 0 0 1 2 2 2
  spline S194 degree 2 poles (-12.0797, 57.2056) (-12.0768, 57.0205) (-11.8902, 56.5939) (-11.7656, 56.3852) knots 0 0 0 1 2 2 2
  spline S195 degree 2 poles (-11.7656, 56.3852) (-11.6186, 56.1388) (-11.0863, 55.5505) (-10.7575, 55.2938) knots 0 0 0 1 2 2 2
  line L159 (-10.7575, 55.2938) -> (-10.7326, 55.252)
  line L160 (-10.7326, 55.252) -> (-11.3964, 54.8558)
  spline S196 degree 2 poles (-11.3964, 54.8558) (-11.5636, 55.0221) (-12.13, 55.6864) (-12.3467, 56.0496) knots 0 0 0 1 2 2 2
  spline S197 degree 2 poles (-12.3467, 56.0496) (-12.6059, 56.4839) (-12.8395, 57.1598) (-12.8212, 57.4992) knots 0 0 0 1 2 2 2
  spline S198 degree 2 poles (-12.8212, 57.4992) (-12.7996, 57.8235) (-12.4314, 58.3546) (-12.0682, 58.5714) knots 0 0 0 1 2 2 2
  line L161 (-12.0682, 58.5714) -> (-9.4253, 60.1488)
  line L162 (-9.4253, 60.1488) -> (-8.9992, 59.4348)
  line L163 (-8.9992, 59.4348) -> (-9.4084, 59.1906)
  line L164 (-9.9511, 58.8667) -> (-11.0242, 58.2263)
  spline S199 degree 2 poles (-11.0242, 58.2263) (-10.8513, 57.9841) (-10.3168, 57.2498) (-10.1055, 57.0475) knots 0 0 0 1 2 2 2
  spline S200 degree 2 poles (-10.1055, 57.0475) (-9.8567, 56.811) (-9.3051, 56.6363) (-9.0128, 56.8107) knots 0 0 0 1 2 2 2
  spline S201 degree 2 poles (-9.0128, 56.8107) (-8.6788, 57.01) (-8.5848, 57.621) (-8.8216, 58.0177) knots 0 0 0 1 2 2 2
  spline S202 degree 2 poles (-8.8216, 58.0177) (-9.0234, 58.3559) (-9.6129, 58.7458) (-9.9511, 58.8667) knots 0 0 0 1 2 2 2
  line L165 (-16.117, 60.5547) -> (-16.0946, 60.5171)
  spline S203 degree 2 poles (-16.0946, 60.5171) (-16.0707, 60.4011) (-15.9148, 60.0072) (-15.8326, 59.8694) knots 0 0 0 1 2 2 2
  spline S204 degree 2 poles (-15.8326, 59.8694) (-15.561, 59.4143) (-14.9643, 59.2495) (-14.48, 59.5385) knots 0 0 0 1 2 2 2
  line L166 (-14.48, 59.5385) -> (-14.3506, 59.6158)
  line L167 (-14.3506, 59.6158) -> (-15.0582, 60.8015)
  line L168 (-15.0582, 60.8015) -> (-14.5196, 61.123)
  line L169 (-14.5196, 61.123) -> (-13.8244, 59.9581)
  line L170 (-13.8244, 59.9581) -> (-10.4968, 61.9441)
  line L171 (-10.4968, 61.9441) -> (-10.0707, 61.2302)
  line L172 (-10.0707, 61.2302) -> (-13.3983, 59.2441)
  line L173 (-13.3983, 59.2441) -> (-13.1093, 58.7598)
  line L174 (-13.1093, 58.7598) -> (-13.6478, 58.4384)
  line L175 (-13.6478, 58.4384) -> (-13.9369, 58.9227)
  line L176 (-13.9369, 58.9227) -> (-14.0663, 58.8454)
  spline S205 degree 2 poles (-14.0663, 58.8454) (-14.7594, 58.4318) (-15.9269, 58.7372) (-16.3381, 59.4261) knots 0 0 0 1 2 2 2
  spline S206 degree 2 poles (-16.3381, 59.4261) (-16.4552, 59.6223) (-16.6469, 60.0289) (-16.714, 60.1983) knots 0 0 0 1 2 2 2
  line L177 (-16.714, 60.1983) -> (-16.117, 60.5547)
  line L178 (-17.5972, 63.0347) -> (-17.5747, 62.9971)
  spline S207 degree 2 poles (-17.5747, 62.9971) (-17.5508, 62.8812) (-17.395, 62.4872) (-17.3127, 62.3494) knots 0 0 0 1 2 2 2
  spline S208 degree 2 poles (-17.3127, 62.3494) (-17.0411, 61.8943) (-16.4445, 61.7295) (-15.9601, 62.0186) knots 0 0 0 1 2 2 2
  line L179 (-15.9601, 62.0186) -> (-15.8307, 62.0958)
  line L180 (-15.8307, 62.0958) -> (-16.5384, 63.2816)
  line L181 (-16.5384, 63.2816) -> (-15.9998, 63.603)
  line L182 (-15.9998, 63.603) -> (-15.3046, 62.4381)
  line L183 (-15.3046, 62.4381) -> (-11.977, 64.4242)
  line L184 (-11.977, 64.4242) -> (-11.5509, 63.7102)
  line L185 (-11.5509, 63.7102) -> (-14.8785, 61.7242)
  line L186 (-14.8785, 61.7242) -> (-14.5894, 61.2399)
  line L187 (-14.5894, 61.2399) -> (-15.128, 60.9184)
  line L188 (-15.128, 60.9184) -> (-15.4171, 61.4027)
  line L189 (-15.4171, 61.4027) -> (-15.5465, 61.3255)
  spline S209 degree 2 poles (-15.5465, 61.3255) (-16.2396, 60.9118) (-17.4071, 61.2173) (-17.8183, 61.9062) knots 0 0 0 1 2 2 2
  spline S210 degree 2 poles (-17.8183, 61.9062) (-17.9354, 62.1024) (-18.1271, 62.5089) (-18.1942, 62.6784) knots 0 0 0 1 2 2 2
  line L190 (-18.1942, 62.6784) -> (-17.5972, 63.0347)
  spline S211 degree 2 poles (-14.8082, 68.2382) (-14.6974, 68.1854) (-14.3143, 68.0177) (-14.1694, 67.9173) knots 0 0 0 1 2 2 2
  spline S212 degree 2 poles (-14.1694, 67.9173) (-13.9654, 67.7843) (-13.6576, 67.4867) (-13.4682, 67.1694) knots 0 0 0 1 2 2 2
  spline S213 degree 2 poles (-13.4682, 67.1694) (-13.3112, 66.9064) (-13.2092, 66.3274) (-13.2648, 66.0507) knots 0 0 0 1 2 2 2
  spline S214 degree 2 poles (-13.2648, 66.0507) (-13.3213, 65.7848) (-13.6668, 65.3012) (-13.9257, 65.1467) knots 0 0 0 1 2 2 2
  spline S215 degree 2 poles (-13.9257, 65.1467) (-14.3265, 64.9074) (-15.1161, 64.9401) (-15.5207, 65.248) knots 0 0 0 1 2 2 2
  spline S216 degree 2 poles (-15.5207, 65.248) (-15.8828, 65.5131) (-16.5761, 66.4187) (-16.9417, 66.9649) knots 0 0 0 1 2 2 2
  line L191 (-16.9417, 66.9649) -> (-17.067, 66.8901)
  spline S217 degree 2 poles (-17.067, 66.8901) (-17.2924, 66.7556) (-17.4825, 66.4383) (-17.4796, 66.2532) knots 0 0 0 1 2 2 2
  spline S218 degree 2 poles (-17.4796, 66.2532) (-17.4767, 66.068) (-17.29, 65.6415) (-17.1655, 65.4327) knots 0 0 0 1 2 2 2
  spline S219 degree 2 poles (-17.1655, 65.4327) (-17.0184, 65.1864) (-16.4861, 64.5981) (-16.1574, 64.3414) knots 0 0 0 1 2 2 2
  line L192 (-16.1574, 64.3414) -> (-16.1324, 64.2996)
  line L193 (-16.1324, 64.2996) -> (-16.7963, 63.9034)
  spline S220 degree 2 poles (-16.7963, 63.9034) (-16.9635, 64.0697) (-17.5298, 64.734) (-17.7466, 65.0972) knots 0 0 0 1 2 2 2
  spline S221 degree 2 poles (-17.7466, 65.0972) (-18.0058, 65.5314) (-18.2393, 66.2074) (-18.221, 66.5468) knots 0 0 0 1 2 2 2
  spline S222 degree 2 poles (-18.221, 66.5468) (-18.1994, 66.8711) (-17.8313, 67.4022) (-17.468, 67.619) knots 0 0 0 1 2 2 2
  line L194 (-17.468, 67.619) -> (-14.8252, 69.1964)
  line L195 (-14.8252, 69.1964) -> (-14.3991, 68.4824)
  line L196 (-14.3991, 68.4824) -> (-14.8082, 68.2382)
  line L197 (-15.351, 67.9143) -> (-16.424, 67.2739)
  spline S223 degree 2 poles (-16.424, 67.2739) (-16.2511, 67.0316) (-15.7167, 66.2974) (-15.5053, 66.0951) knots 0 0 0 1 2 2 2
  spline S224 degree 2 poles (-15.5053, 66.0951) (-15.2566, 65.8586) (-14.705, 65.6838) (-14.4127, 65.8583) knots 0 0 0 1 2 2 2
  spline S225 degree 2 poles (-14.4127, 65.8583) (-14.0787, 66.0576) (-13.9847, 66.6686) (-14.2214, 67.0653) knots 0 0 0 1 2 2 2
  spline S226 degree 2 poles (-14.2214, 67.0653) (-14.4233, 67.4034) (-15.0127, 67.7934) (-15.351, 67.9143) knots 0 0 0 1 2 2 2
  point P0 (0, 0)
  constraints: 2 other
extrude "Extrusion2" cut sketch "Sketch2" against normal blind 5
equation "\"d5\" = 0.8 * d2"
body "Solid1"
